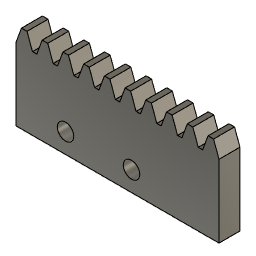
Top part assembly v19 (Autodesk Fusion 360 archive; units mm, degrees)
design "Mod 2 Rack Gear"
Autodesk Fusion 360 part; units mm, degrees
note: some values were not read from the file. Set by a fixed rule: which sketch regions a step uses.
sketch "Sketch1" plane through (0, 0, 0) normal (0, 0, 1) x (1, 0, 0) in component "Component"
  line L0 (0, 0) -> (1.6379, 4.5)
  line L1 (3.3236, 4.5) -> (4.9614, 0)
  line L2 (1.6379, 4.5) -> (3.3236, 4.5)
  line L3 (0, 0) -> (0, -10)
  line L4 (0, -10) -> (4.9614, -10)
  line L5 (4.9614, -10) -> (4.9614, 0)
  line L6 (2.1819, 0) -> (100, 0)
  line L7 (0, 0, 0) -> (0, 0, 6.35)
sketch "Sketch2" plane through (0, 0, 0) normal (0, 0, 1) x (1, 0, 0) in component "Component"
  line L0 (0, 0) -> (61.5101, 0)
  line L1 (0, 0) -> (0, -10)
  line L2 (0, -10) -> (61.5101, -10)
  line L3 (61.5101, -10) -> (61.5101, 0)
sweep "Sweep1" add kept parallel profiles "Sketch1" path "Sketch1" along L7 section 1 makes body 1 in component "Component"
pattern_path "PathPattern1" count 10 spacing 6.2832 from (2.1819, 0, 0) path "Sketch1" along L6 of "Sweep1" makes body 2 makes body 3 makes body 4 makes body 5 makes body 6 makes body 7 makes body 8 makes body 9 makes body 10 in component "Component"
extrude "Extrude1" add sketch "Sketch2" along normal blind 6.35 bodies 1 2 3 4 5 6 7 8 9 10 in component "Component"
move_body "Move1" bodies 1 to x (1, 0, 0) y (0, 0, 1) z (0, -1, 0) at (0, -10, 10) in component "Component"
sketch "Sketch3" plane through (0, 0, 0) normal (0, 0, 1) x (1, 0, 0) in component "Component"
  line L0 (0, 0) -> (49.9131, 0) construction
  line L1 (49.9131, 0) -> (49.9131, 3) construction
  line L2 (49.9131, 3) -> (0, 3) construction
  line L3 (0, 3) -> (0, 0) construction
  constraint perpendicular L0 L1
  constraint parallel L0 L2
  constraint parallel L1 L3
extrude "Extrude3" add 1 faces at (20.5034, -14.2333, 0) along direction (0, 0, -1) blind 12 on bodies 1 bodies 1 in component "Component"
sketch "Sketch1 (2)" plane through (0, -16.35, 0) normal (0, -1, 0) x (1, 0, 0)
  line L0 (55.2269, 10) -> (53.5891, 14.5)
  line L1 (53.5891, 14.5) -> (51.9033, 14.5)
  line L2 (51.9033, 14.5) -> (50.2655, 10)
  line L3 (50.2655, 10) -> (48.9437, 10)
  line L4 (48.9437, 10) -> (47.3059, 14.5)
  line L5 (47.3059, 14.5) -> (45.6202, 14.5)
  line L6 (45.6202, 14.5) -> (43.9823, 10)
  line L7 (43.9823, 10) -> (42.6606, 10)
  line L8 (42.6606, 10) -> (41.0227, 14.5)
  line L9 (41.0227, 14.5) -> (39.337, 14.5)
  line L10 (39.337, 14.5) -> (37.6991, 10)
  line L11 (37.6991, 10) -> (36.3774, 10)
  line L12 (36.3774, 10) -> (34.7395, 14.5)
  line L13 (34.7395, 14.5) -> (33.0538, 14.5)
  line L14 (33.0538, 14.5) -> (31.4159, 10)
  line L15 (31.4159, 10) -> (30.0942, 10)
  line L16 (30.0942, 10) -> (28.4563, 14.5)
  line L17 (28.4563, 14.5) -> (26.7706, 14.5)
  line L18 (26.7706, 14.5) -> (25.1327, 10)
  line L19 (25.1327, 10) -> (23.811, 10)
  line L20 (23.811, 10) -> (22.1731, 14.5)
  line L21 (22.1731, 14.5) -> (20.4874, 14.5)
  line L22 (20.4874, 14.5) -> (18.8496, 10)
  line L23 (18.8496, 10) -> (17.5278, 10)
  line L24 (17.5278, 10) -> (15.8899, 14.5)
  line L25 (15.8899, 14.5) -> (14.2042, 14.5)
  line L26 (14.2042, 14.5) -> (12.5664, 10)
  line L27 (12.5664, 10) -> (11.2446, 10)
  line L28 (11.2446, 10) -> (9.6068, 14.5)
  line L29 (9.6068, 14.5) -> (7.9211, 14.5)
  line L30 (7.9211, 14.5) -> (6.2832, 10)
  line L31 (6.2832, 10) -> (4.9614, 10)
  line L32 (4.9614, 10) -> (3.3236, 14.5)
  line L33 (3.3236, 14.5) -> (1.6379, 14.5)
  line L34 (1.6379, 14.5) -> (0, 10)
  line L35 (0, 10) -> (0, -12)
  line L36 (61.5101, -12) -> (61.5101, 10)
  line L37 (61.5101, 10) -> (59.8722, 14.5)
  line L38 (59.8722, 14.5) -> (58.1865, 14.5)
  line L39 (58.1865, 14.5) -> (56.5487, 10)
  line L40 (56.5487, 10) -> (55.2269, 10)
  line L41 (0, -6) -> (61.5101, -6) construction
  line L42 (30.7551, -11.3817) -> (30.7551, -6) construction
  circle A0 centre (15, -6) radius 2.5
  circle A1 centre (35, -6) radius 2.5
  line L43 (0, -12) -> (61.5101, -12)
  point P0 (30.7551, -11.3817)
  dimension "d11" = 5
  dimension "d12" = 5
  dimension "d13" = 20
  dimension "d17" = 6
  dimension "d18" = 15
  constraint coincident P0 L42.start
  constraint midpoint L41 L42.end
  constraint coincident L41 A0.centre
  constraint coincident L41 A1.centre
  constraint horizontal L41
  constraint coincident L36 L41.end
  constraint coincident L35 L41.start
  measures "d11" diameter of A0
  measures "d12" diameter of A1
  measures "d13" distance of A0.centre A1.centre
  measures "d17" distance of L41 L43
  measures "d18" horizontal distance of L35.end A0.centre
extrude "Extrude2" cut sketch "Sketch1 (2)" against normal through all contours A0 | A1 bodies 1 in component "Component"
component "Component" placed x (1, 0, 0) y (0, 1, 0) z (0, 0, 1) at (0, 0, 0)

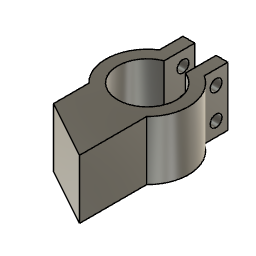
design "clamp"
Autodesk Fusion 360 part; units mm, degrees
sketch "Sketch1" plane through (0, 0, 0) normal (0, 0, 1) x (1, 0, 0)
  circle A0 centre (0, 0) radius 12.5
  circle A1 centre (0, 0) radius 17.5
  line L0 (-9.525, 14.6807) -> (9.525, 14.6807)
  line L1 (-4.525, 11.6522) -> (-9.525, 11.6522)
  line L2 (-9.525, 11.6522) -> (-9.525, 24.6807)
  line L3 (-9.525, 24.6807) -> (-4.525, 24.6807)
  line L4 (-4.525, 24.6807) -> (-4.525, 11.6522)
  line L5 (4.525, 11.6522) -> (9.525, 11.6522)
  line L6 (9.525, 11.6522) -> (9.525, 24.6807)
  line L7 (9.525, 24.6807) -> (4.525, 24.6807)
  line L8 (4.525, 24.6807) -> (4.525, 11.6522)
  line L9 (0.0006, -27.5) -> (12.2475, -27.5)
  line L10 (12.2475, -27.5) -> (12.2475, -12.5)
  line L11 (12.2475, -12.5) -> (0.0006, -12.5)
  line L12 (0.0006, -12.5) -> (0.0006, -27.5)
  line L13 (-12.2462, -27.5) -> (-12.2462, -12.5)
  line L14 (0.0006, -27.5) -> (-12.2462, -27.5)
  line L15 (-12.2462, -12.5) -> (0.0006, -12.5)
  line L16 (12.2475, -27.5) -> (12.2475, -41)
  line L17 (12.2475, -41) -> (-12.2462, -27.5)
  dimension "d1" = 25
  dimension "d2" = 35
  dimension "d3" = 19.05
  dimension "d4" = 10
  dimension "d5" = 5
  dimension "d6" = 5
  dimension "d7" = 10
  dimension "d18" = 12.2468
  dimension "d19" = 15
  dimension "d27" = 13.5
  constraint coincident A0.centre A1.centre
  constraint coincident A1 L0.start
  constraint coincident A1 L0.end
  constraint horizontal L0
  constraint horizontal L1
  constraint vertical L2
  constraint horizontal L3
  constraint vertical L4
  constraint coincident A0 L1.start
  constraint horizontal L5
  constraint vertical L6
  constraint horizontal L7
  constraint vertical L8
  constraint coincident A0 L5.start
  constraint coincident L0.end L6
  constraint coincident L0.start L2
  constraint horizontal L9
  constraint vertical L10
  constraint horizontal L11
  constraint vertical L12
  constraint coincident A1 L10.end
  constraint coincident A0 L11.end
  constraint symmetric L9.start L12 L14.start
  constraint symmetric L9.end L12 L13.start
  constraint symmetric L10.end L12 L13.end
  constraint symmetric L11.end L12 L15.end
  constraint perpendicular L9 L16
  measures "d1" diameter of A0
  measures "d2" diameter of A1
  measures "d3" distance of L0.start L0.end
  measures "d4" distance of L0.start L2.end
  measures "d5" distance of L2.end L3.end
  measures "d6" distance of L5.start L5.end
  measures "d7" distance of L0.end L6.end
  measures "d18" distance of L9.start L9.end
  measures "d19" distance of L9.end L10.end
  measures "d27" distance of L9.end L16.end
extrude "Extrude1" add sketch "Sketch1" along normal blind 25 contours A0 A1 L5 L6 L11 | L0 L5 L6 L8 | A0 A1 L1 L2 L15 | A1 L11 L12 | A1 L12 L15 | L0 L1 L2 L4 | A1 L0 L8 | A1 L9 L10 L12 | A1 L12 L13 L14 | A1 L0 L4 | A1 L6 L7 L8 | L9 L14 L16 L17 | A1 L2 L3 L4
hole "Hole1" at (9.525, 19.6807, 19) direction (-1, 0, 0) diameter 5 depth 20 tip angle 180
hole "Hole2" at (-9.525, 19.6807, 6) direction (1, 0, 0) diameter 5 depth 20 tip angle 180
equation "d6 = d5"
equation "d7 = d4"

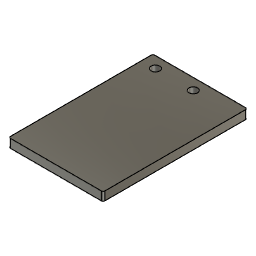
design "supporting part"
Autodesk Fusion 360 part; units mm, degrees
sketch "草图1" plane through (0, 0, 0) normal (0, 0, 1) x (1, 0, 0)
  line L0 (-27.5, -48) -> (27.5, -48)
  line L1 (27.5, -48) -> (27.5, -132)
  line L2 (27.5, -132) -> (-27.5, -132)
  line L3 (-27.5, -48) -> (-27.5, -132)
  line L4 (0, 1.75) -> (0, 22.5)
  circle A0 centre (-19.5, -54.5) radius 2.5
  circle A1 centre (2.5, -54.5) radius 2.5
  dimension "d1" = 55
  dimension "d2" = 55
  dimension "d3" = 84
  dimension "d4" = 48
  dimension "d13" = 5
  dimension "d14" = 5
  dimension "d15" = 22
  dimension "d16" = 6.5
  dimension "d17" = 8
  constraint horizontal L0
  constraint perpendicular L0 L1
  constraint perpendicular L1 L2
  constraint symmetric L1.end L2.end L4
  constraint horizontal A0.centre A1.centre
  measures "d1" distance of L0.start L0.end
  measures "d2" distance of L1.end L2.end
  measures "d3" distance of L0.end L1.end
  measures "d4" vertical distance of origin L0.start
  measures "d13" diameter of A0
  measures "d14" diameter of A1
  measures "d15" horizontal distance of A0.centre A1.centre
  measures "d16" distance of L0 A0.centre
  measures "d17" distance of L3 A0.centre
extrude "拉伸1" add sketch "草图1" along normal blind 5
fillet "Fillet1" radius 1 4 edges at (-27.5, -48, 2.5) (27.5, -48, 2.5) (27.5, -132, 2.5) (-27.5, -132, 2.5)
equation "d14 = d13"
